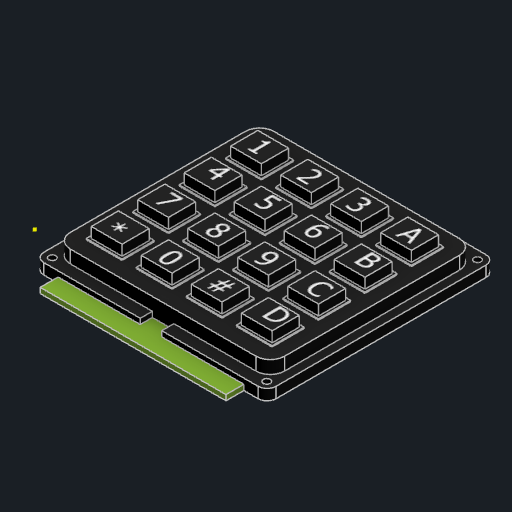
# Autodesk Inventor part: keypad
Saved by Autodesk Inventor 2023 (Build 270158000, 158)
## iProperties
Created: 2021-01-26
Part Number: keypad
Material: Generic
Document SubType Name: Modeling
Designer: Diego
Density: 1 g/cm^3
Appearance: Default
Author: Diego
Autodesk Inventor part; units mm, degrees
ref_plane "YZ Plane" through (0, 0, 0) normal (1, 0, 0) x (0, 1, 0)
ref_plane "XZ Plane" through (0, 0, 0) normal (0, 1, 0) x (-1, 0, 0)
ref_plane "XY Plane" through (0, 0, 0) normal (0, 0, 1) x (1, 0, 0)
sketch "Sketch1" plane through (0, 0, 0) normal (0, 0, 1) x (1, 0, 0)
  line L0 (0, 0) -> (65, 0)
  line L1 (65, 0) -> (65, 63.8)
  line L2 (65, 63.8) -> (0, 63.8)
  line L3 (0, 63.8) -> (0, 0)
  dimension "d0" = 65
  dimension "d1" = 63.8
  constraints: 8 end point, 2 parallel, 1 horizontal, 1 perpendicular
  measures "d0" distance of L2.end L1.end
  measures "d1" distance of L1.end L0.end
extrude "Extrusion1" add sketch "Sketch1" along normal blind 3
fillet "Fillet1" radius 2.5 4 edges at (65, 63.8, 1.5) (0, 63.8, 1.5) (65, 0, 1.5) (0, 0, 1.5)
sketch "Sketch2" plane through (0, 0, 3) normal (0, 0, 1) x (1, 0, 0)
  line L0 (2.5, 3.4) -> (62.5, 3.4)
  line L1 (62.5, 3.4) -> (62.5, 60.4)
  line L2 (62.5, 60.4) -> (2.5, 60.4)
  line L3 (2.5, 60.4) -> (2.5, 3.4)
  line L4 (2.5, 0) -> (62.5, 0) projected
  line L5 (0, 61.3) -> (0, 2.5) projected
  point P0 (0, 0)
  dimension "d5" = 60
  dimension "d6" = 57
  dimension "d7" = 3.4
  dimension "d8" = 2.5
  constraints: 8 end point, 2 parallel, 1 horizontal, 1 perpendicular
  measures "d5" distance of L2.end L1.end
  measures "d6" distance of L1.end L0.end
  measures "d7" distance between parallel lines of L4 L0
  measures "d8" distance between parallel lines of L5 L3
extrude "Extrusion2" add sketch "Sketch2" along normal blind 3.6
fillet "Fillet2" radius 4 4 edges at (62.5, 60.4, 4.8) (2.5, 60.4, 4.8) (62.5, 3.4, 4.8) (2.5, 3.4, 4.8)
sketch "Sketch3" plane through (0, 0, 6.6) normal (0, 0, 1) x (1, 0, 0)
  line L0 (6.5, 55.9) -> (16.5, 55.9)
  line L1 (16.5, 55.9) -> (16.5, 46.9)
  line L2 (16.5, 46.9) -> (6.5, 46.9)
  line L3 (6.5, 46.9) -> (6.5, 55.9)
  line L4 (6.5, 42.9) -> (16.5, 42.9)
  line L5 (16.5, 42.9) -> (16.5, 33.9)
  line L6 (16.5, 33.9) -> (6.5, 33.9)
  line L7 (6.5, 33.9) -> (6.5, 42.9)
  line L8 (6.5, 29.9) -> (16.5, 29.9)
  line L9 (16.5, 29.9) -> (16.5, 20.9)
  line L10 (16.5, 20.9) -> (6.5, 20.9)
  line L11 (6.5, 20.9) -> (6.5, 29.9)
  line L12 (6.5, 16.9) -> (16.5, 16.9)
  line L13 (16.5, 16.9) -> (16.5, 7.9)
  line L14 (16.5, 7.9) -> (6.5, 7.9)
  line L15 (6.5, 7.9) -> (6.5, 16.9)
  line L16 (20.5, 55.9) -> (30.5, 55.9)
  line L17 (30.5, 55.9) -> (30.5, 46.9)
  line L18 (30.5, 46.9) -> (20.5, 46.9)
  line L19 (20.5, 46.9) -> (20.5, 55.9)
  line L20 (20.5, 42.9) -> (30.5, 42.9)
  line L21 (30.5, 42.9) -> (30.5, 33.9)
  line L22 (30.5, 33.9) -> (20.5, 33.9)
  line L23 (20.5, 33.9) -> (20.5, 42.9)
  line L24 (20.5, 29.9) -> (30.5, 29.9)
  line L25 (30.5, 29.9) -> (30.5, 20.9)
  line L26 (30.5, 20.9) -> (20.5, 20.9)
  line L27 (20.5, 20.9) -> (20.5, 29.9)
  line L28 (20.5, 16.9) -> (30.5, 16.9)
  line L29 (30.5, 16.9) -> (30.5, 7.9)
  line L30 (30.5, 7.9) -> (20.5, 7.9)
  line L31 (20.5, 7.9) -> (20.5, 16.9)
  line L32 (34.5, 55.9) -> (44.5, 55.9)
  line L33 (44.5, 55.9) -> (44.5, 46.9)
  line L34 (44.5, 46.9) -> (34.5, 46.9)
  line L35 (34.5, 46.9) -> (34.5, 55.9)
  line L36 (34.5, 42.9) -> (44.5, 42.9)
  line L37 (44.5, 42.9) -> (44.5, 33.9)
  line L38 (44.5, 33.9) -> (34.5, 33.9)
  line L39 (34.5, 33.9) -> (34.5, 42.9)
  line L40 (34.5, 29.9) -> (44.5, 29.9)
  line L41 (44.5, 29.9) -> (44.5, 20.9)
  line L42 (44.5, 20.9) -> (34.5, 20.9)
  line L43 (34.5, 20.9) -> (34.5, 29.9)
  line L44 (34.5, 16.9) -> (44.5, 16.9)
  line L45 (44.5, 16.9) -> (44.5, 7.9)
  line L46 (44.5, 7.9) -> (34.5, 7.9)
  line L47 (34.5, 7.9) -> (34.5, 16.9)
  line L48 (48.5, 55.9) -> (58.5, 55.9)
  line L49 (58.5, 55.9) -> (58.5, 46.9)
  line L50 (58.5, 46.9) -> (48.5, 46.9)
  line L51 (48.5, 46.9) -> (48.5, 55.9)
  line L52 (48.5, 42.9) -> (58.5, 42.9)
  line L53 (58.5, 42.9) -> (58.5, 33.9)
  line L54 (58.5, 33.9) -> (48.5, 33.9)
  line L55 (48.5, 33.9) -> (48.5, 42.9)
  line L56 (48.5, 29.9) -> (58.5, 29.9)
  line L57 (58.5, 29.9) -> (58.5, 20.9)
  line L58 (58.5, 20.9) -> (48.5, 20.9)
  line L59 (48.5, 20.9) -> (48.5, 29.9)
  line L60 (48.5, 16.9) -> (58.5, 16.9)
  line L61 (58.5, 16.9) -> (58.5, 7.9)
  line L62 (58.5, 7.9) -> (48.5, 7.9)
  line L63 (48.5, 7.9) -> (48.5, 16.9)
  line L64 (2.5, 56.4) -> (2.5, 7.4) projected
  line L65 (58.5, 60.4) -> (6.5, 60.4) projected
  point P0 (0, 0)
  dimension "d12" = 10
  dimension "d13" = 9
  dimension "d16" = 13
  dimension "d19" = 14
  dimension "d22" = 52
  dimension "d23" = 4
  dimension "d24" = 48
  dimension "d25" = 22
  dimension "d26" = 24
  dimension "d27" = 4.5
  constraints: 128 end point, 2 collinear, 2 horizontal, 2 parallel, 1 perpendicular, 1 vertical, 118 other
  measures "d12" distance of L1.end L2.end
  measures "d13" distance of L0.end L1.end
  measures "d16" distance of L0.start L4.start
  measures "d19" distance of L0.start L16.start
  measures "d22" distance between parallel lines of L3 L49
  measures "d23" distance between parallel lines of L64 L3
  measures "d24" distance between parallel lines of L14 L0
  measures "d25" distance between parallel lines of L4 L10
  measures "d26" distance between parallel lines of L33 L19
  measures "d27" distance between parallel lines of L65 L0
extrude "Extrusion3" add sketch "Sketch3" along normal blind 0.3
sketch "Sketch4" plane through (0, 0, 6.9) normal (0, 0, 1) x (1, 0, 0)
  line L0 (7.2, 47.6) -> (15.8, 47.6)
  line L1 (15.8, 47.6) -> (15.8, 55.2)
  line L2 (15.8, 55.2) -> (7.2, 55.2)
  line L3 (7.2, 55.2) -> (7.2, 47.6)
  line L4 (6.5, 55.9) -> (6.5, 46.9) projected
  line L5 (6.5, 46.9) -> (16.5, 46.9) projected
  point P0 (0, 0)
  dimension "d30" = 8.6
  dimension "d31" = 7.6
  dimension "d32" = 0.7
  dimension "d33" = 0.7
  constraints: 8 end point, 2 parallel, 1 horizontal, 1 perpendicular
  measures "d30" distance of L2.end L1.end
  measures "d31" distance of L1.end L0.end
  measures "d32" distance between parallel lines of L4 L3
  measures "d33" distance between parallel lines of L5 L0
extrude "Extrusion4" add sketch "Sketch4" along normal blind 2.9
pattern_linear "Rectangular Pattern1" count 4 spacing 13 along (0, -1, 0) count 4 spacing 14 along (1, 0, 0) of "Extrusion4"
sketch "Sketch5" plane through (0, 0, 3) normal (0, 0, 1) x (1, 0, 0)
  line L0 (2.5, 0) -> (62.5, 0) projected
  line L1 (29.5, 3.4) -> (35.5, 3.4)
  line L2 (35.5, 3.4) -> (35.5, 0)
  line L3 (35.5, 0) -> (29.5, 0)
  line L4 (29.5, 0) -> (29.5, 3.4)
  line L5 (6.5, 3.4) -> (58.5, 3.4) projected
  line L6 (65, 2.5) -> (65, 61.3) projected
  line L7 (0, 61.3) -> (0, 2.5) projected
  point P0 (0, 0)
  dimension "d42" = 6
  dimension "d43" = 0
  dimension "d44" = 29.5
  dimension "d45" = 29.5
  constraints: 8 end point, 2 parallel, 1 horizontal, 1 perpendicular, 1 point on line
  measures "d42" distance of L2.end L3.end
  measures "d43" distance between parallel lines of L5 L1
  measures "d44" distance between parallel lines of L6 L2
  measures "d45" distance between parallel lines of L7 L4
extrude "Extrusion5" cut sketch "Sketch5" against normal through all
sketch "Sketch6" plane through (0, 0, 0) normal (0, 0, -1) x (-1, 0, 0)
  line L0 (-6.5, 7.9) -> (-6.5, 16.9) projected
  line L1 (-58.5, 16.9) -> (-58.5, 7.9) projected
  line L2 (-6.5, 3.4) -> (-58.5, 3.4) projected
  line L3 (-58.5, 3.4) -> (-6.5, 3.4)
  line L4 (-6.5, 3.4) -> (-6.5, -5)
  line L5 (-6.5, -5) -> (-58.5, -5)
  line L6 (-58.5, -5) -> (-58.5, 3.4)
  line L7 (-2.5, 0) -> (-29.5, 0) projected
  point P0 (0, 0)
  dimension "d48" = 5
  constraints: 8 end point, 2 parallel, 1 horizontal, 1 perpendicular
  measures "d48" distance between parallel lines of L5 L7
extrude "Extrusion6" add sketch "Sketch6" against normal blind 1.5
sketch "Sketch7" plane through (0, 0, 3) normal (0, 0, 1) x (1, 0, 0)
  line L0 (2.5, 2.4) -> (62.5, 2.4)
  line L1 (62.5, 2.4) -> (62.5, 61.4)
  line L2 (62.5, 61.4) -> (2.5, 61.4)
  line L3 (2.5, 61.4) -> (2.5, 2.4)
  line L4 (65, 2.5) -> (65, 61.3) projected
  line L5 (62.5, 63.8) -> (2.5, 63.8) projected
  point P0 (0, 0)
  dimension "d51" = 60
  dimension "d52" = 59
  dimension "d53" = 2.5
  dimension "d54" = 2.4
  constraints: 8 end point, 2 parallel, 1 horizontal, 1 perpendicular
  measures "d51" distance of L2.end L1.end
  measures "d52" distance of L1.end L0.end
  measures "d53" distance between parallel lines of L4 L1
  measures "d54" distance between parallel lines of L5 L2
hole "Hole1" at (62.5, 61.4, 3) at (62.5, 2.4, 3) at (2.5, 2.4, 3) at (2.5, 61.4, 3) direction (0, 0, -1) diameter 2 end through all
sketch "Sketch9" plane through (0, 0, 9.8) normal (0, 0, 1) x (1, 0, 0)
  line L0 (9.6076, 54.1981) -> (13.48, 54.1981) construction
  line L1 (13.48, 54.1981) -> (13.48, 49.6601) construction
  line L2 (13.48, 49.6601) -> (9.6076, 49.6601) construction
  line L3 (9.6076, 49.6601) -> (9.6076, 54.1981) construction
  line L4 (23.8211, 53.9737) -> (27.6934, 53.9737) construction
  line L5 (27.6934, 53.9737) -> (27.6934, 49.4357) construction
  line L6 (27.6934, 49.4357) -> (23.8211, 49.4357) construction
  line L7 (23.8211, 49.4357) -> (23.8211, 53.9737) construction
  line L8 (37.5104, 54.003) -> (41.3828, 54.003) construction
  line L9 (41.3828, 54.003) -> (41.3828, 49.465) construction
  line L10 (41.3828, 49.465) -> (37.5104, 49.465) construction
  line L11 (37.5104, 49.465) -> (37.5104, 54.003) construction
  line L12 (51.8676, 49.4469) -> (51.8676, 53.9849) construction
  line L13 (51.8676, 53.9849) -> (55.74, 53.9849) construction
  line L14 (55.74, 53.9849) -> (55.74, 49.4469) construction
  line L15 (55.74, 49.4469) -> (51.8676, 49.4469) construction
  line L16 (9.9297, 41.8514) -> (13.802, 41.8514) construction
  line L17 (13.802, 41.8514) -> (13.802, 37.3134) construction
  line L18 (13.802, 37.3134) -> (9.9297, 37.3134) construction
  line L19 (9.9297, 37.3134) -> (9.9297, 41.8514) construction
  line L20 (24.1431, 37.0889) -> (24.1431, 41.627) construction
  line L21 (24.1431, 41.627) -> (28.0155, 41.627) construction
  line L22 (28.0155, 41.627) -> (28.0155, 37.0889) construction
  line L23 (28.0155, 37.0889) -> (24.1431, 37.0889) construction
  line L24 (37.8325, 37.1182) -> (37.8325, 41.6562) construction
  line L25 (37.8325, 41.6562) -> (41.7049, 41.6562) construction
  line L26 (41.7049, 41.6562) -> (41.7049, 37.1182) construction
  line L27 (41.7049, 37.1182) -> (37.8325, 37.1182) construction
  line L28 (52.1897, 37.1001) -> (52.1897, 41.6381) construction
  line L29 (52.1897, 41.6381) -> (56.0621, 41.6381) construction
  line L30 (56.0621, 41.6381) -> (56.0621, 37.1001) construction
  line L31 (56.0621, 37.1001) -> (52.1897, 37.1001) construction
  line L32 (9.8143, 28.2237) -> (13.6866, 28.2237) construction
  line L33 (13.6866, 28.2237) -> (13.6866, 23.6857) construction
  line L34 (13.6866, 23.6857) -> (9.8143, 23.6857) construction
  line L35 (9.8143, 23.6857) -> (9.8143, 28.2237) construction
  line L36 (24.0277, 23.4613) -> (24.0277, 27.9993) construction
  line L37 (24.0277, 27.9993) -> (27.9001, 27.9993) construction
  line L38 (27.9001, 27.9993) -> (27.9001, 23.4613) construction
  line L39 (27.9001, 23.4613) -> (24.0277, 23.4613) construction
  line L40 (37.7171, 23.4906) -> (37.7171, 28.0286) construction
  line L41 (37.7171, 28.0286) -> (41.5894, 28.0286) construction
  line L42 (41.5894, 28.0286) -> (41.5894, 23.4906) construction
  line L43 (41.5894, 23.4906) -> (37.7171, 23.4906) construction
  line L44 (52.0743, 23.4725) -> (52.0743, 28.0105) construction
  line L45 (52.0743, 28.0105) -> (55.9466, 28.0105) construction
  line L46 (55.9466, 28.0105) -> (55.9466, 23.4725) construction
  line L47 (55.9466, 23.4725) -> (52.0743, 23.4725) construction
  line L48 (9.4563, 9.4122) -> (9.4563, 13.9502) construction
  line L49 (9.4563, 13.9502) -> (13.3287, 13.9502) construction
  line L50 (13.3287, 13.9502) -> (13.3287, 9.4122) construction
  line L51 (13.3287, 9.4122) -> (9.4563, 9.4122) construction
  line L52 (24.0098, 10.2078) -> (24.0098, 14.7459) construction
  line L53 (24.0098, 14.7459) -> (27.8821, 14.7459) construction
  line L54 (27.8821, 14.7459) -> (27.8821, 10.2078) construction
  line L55 (27.8821, 10.2078) -> (24.0098, 10.2078) construction
  line L56 (37.2458, 10.3504) -> (37.2458, 14.8885) construction
  line L57 (37.2458, 14.8885) -> (41.1181, 14.8885) construction
  line L58 (41.1181, 14.8885) -> (41.1181, 10.3504) construction
  line L59 (41.1181, 10.3504) -> (37.2458, 10.3504) construction
  line L60 (52.3964, 11.1257) -> (52.3964, 15.6638) construction
  line L61 (52.3964, 15.6638) -> (56.2687, 15.6638) construction
  line L62 (56.2687, 15.6638) -> (56.2687, 11.1257) construction
  line L63 (56.2687, 11.1257) -> (52.3964, 11.1257) construction
  point P0 (0, 0)
  constraints: 32 other
body "Solid1"
